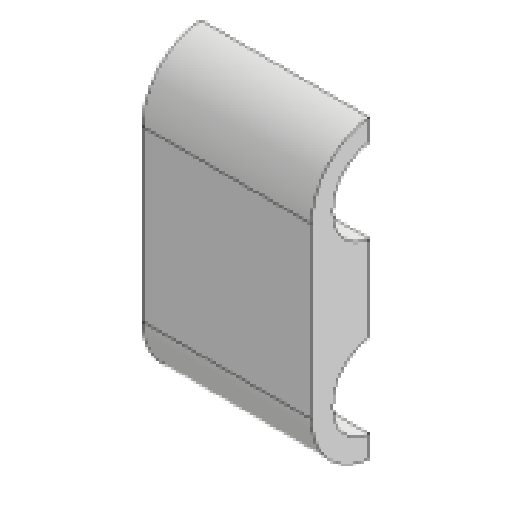
# Autodesk Inventor part: Clamping Part
Saved by Autodesk Inventor 2023 (Build 270158000, 158)
## iProperties
Created: 2022-10-29
Part Number: Clamping Part
Material: Generic
Document SubType Name: Modeling
Designer: deli
Density: 1 g/cm^3
Appearance: Default
Author: deli
Autodesk Inventor part; units mm, degrees
ref_plane "YZ Plane" through (0, 0, 0) normal (1, 0, 0) x (0, 1, 0)
ref_plane "XZ Plane" through (0, 0, 0) normal (0, 1, 0) x (-1, 0, 0)
ref_plane "XY Plane" through (0, 0, 0) normal (0, 0, 1) x (1, 0, 0)
sketch "Sketch1" plane through (0, 0, 0) normal (1, 0, 0) x (0, 1, 0)
  arc A0 (25.612, 42.7998) -> (17.6748, 42.7998) centre (21.6434, 42.2998) ccw
  arc A1 (9.612, 42.7998) -> (1.6748, 42.7998) centre (5.6434, 42.2998) ccw
  arc A2 (27.6225, 42.7998) -> (21.6434, 48.2998) centre (21.6434, 42.2998) ccw
  arc A3 (5.6434, 48.2998) -> (-0.3357, 42.7998) centre (5.6434, 42.2998) ccw
  line L0 (21.6434, 48.2998) -> (5.6434, 48.2998)
  line L1 (27.6225, 42.7998) -> (-0.3357, 42.7998)
  point P0 (0, 0)
  dimension "d0" = 8
  dimension "d1" = 2
  dimension "d2" = 16
  dimension "d3" = 0.5
  constraints: 8 point on circle, 4 centre point, 4 end point, 4 point on line, 2 coincident, 2 equal radius, 2 horizontal, 2 tangent
  measures "d0" diameter of A0
  measures "d1" radial gap between concentric circles of A0 A2
  measures "d2" distance of L0.start L0.end
  measures "d3" distance from line of A1.centre L1
extrude "Extrusion1" add sketch "Sketch1" along normal blind 16 contours A0 L1 A1 A3 L0 A2
sketch "Sketch2" plane through (0, 5.6434, 48.2998) normal (0, 0, 1) x (1, 0, 0)
  line L0 (0, 19.9686) -> (0, 12.0314) construction
  line L1 (16, 16) -> (16, 0) construction
  line L2 (0, 16) -> (16, 0) construction
  circle A0 centre (8, 8) radius 2
  point P0 (0, -5.6434)
  dimension "d6" = 4
  constraints: 2 end point, 2 midpoint, 1 centre point
  measures "d6" diameter of A0
extrude "Extrusion2" cut sketch "Sketch2" against normal blind 16
sketch "Sketch3" plane through (0, 5.6434, 48.2998) normal (0, 0, 1) x (1, 0, 0)
  circle A0 centre (8, 8) radius 2 projected
  circle A1 centre (8, 8) radius 3.75
  point P0 (0, -5.6434)
  dimension "d9" = 7.5
  constraints: 1 centre point, 1 coincident
  measures "d9" diameter of A1
extrude "Extrusion3" cut sketch "Sketch3" against normal blind 4
body "Solid1"
